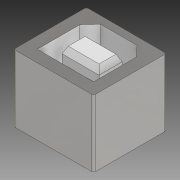
# Autodesk Inventor part: USB B Female Port
Saved by Autodesk Inventor 2016 (Build 200138000, 138)
## iProperties
Created: 2017-10-16
Part Number: USB B Female Port
Material: Steel, Mild
Document SubType Name: Modeling
Designer: admin
Density: 7.85 g/cm^3
Appearance: Semi-Polished
Author: admin
Autodesk Inventor part; units mm, degrees
ref_plane "YZ Plane" through (0, 0, 0) normal (1, 0, 0) x (0, 1, 0)
ref_plane "XZ Plane" through (0, 0, 0) normal (0, 1, 0) x (-1, 0, 0)
ref_plane "XY Plane" through (0, 0, 0) normal (0, 0, 1) x (1, 0, 0)
sketch "Sketch1" plane through (0, 0, 0) normal (0, 0, 1) x (1, 0, 0)
  line L0 (-6.0434, 5.1689) -> (-6.0434, -5.8039) construction
  line L1 (-6.0434, -5.8039) -> (6.0216, -5.8039) construction
  line L2 (6.0216, -5.8039) -> (6.0216, 5.1689) construction
  line L3 (6.0216, 5.1689) -> (-6.0434, 5.1689) construction
  line L4 (-4.2654, -4.0259) -> (4.2436, -4.0259) construction
  line L5 (-4.2654, 2.4003) -> (-4.2654, -4.0259) construction
  line L6 (-2.7795, 4.0259) -> (-4.2654, 2.4003) construction
  line L7 (2.7577, 4.0259) -> (-2.7795, 4.0259) construction
  line L8 (4.2436, 2.4003) -> (2.7577, 4.0259) construction
  line L9 (4.2436, -4.0259) -> (4.2436, 2.4003) construction
  line L10 (-4.2654, -4.0259) -> (4.2436, -4.0259) construction
  line L11 (4.2436, -4.0259) -> (4.2436, 2.4003) construction
  line L12 (4.2436, 2.4003) -> (2.7577, 4.0259) construction
  line L13 (2.7577, 4.0259) -> (-2.7795, 4.0259) construction
  line L14 (-2.7795, 4.0259) -> (-4.2654, 2.4003) construction
  line L15 (-4.2654, 2.4003) -> (-4.2654, -4.0259) construction
  line L16 (1.9887, -1.7399) -> (2.7831, -1.7399) construction
  line L17 (1.9887, -1.8669) -> (1.9887, -1.7399) construction
  line L18 (1.9887, -1.8669) -> (1.0213, -1.8669) construction
  line L19 (1.0213, -1.8669) -> (1.0213, -1.7399) construction
  line L20 (-1.0213, -1.7399) -> (1.0213, -1.7399) construction
  line L21 (-1.0213, -1.8669) -> (-1.0213, -1.7399) construction
  line L22 (-1.0213, -1.8669) -> (-1.9887, -1.8669) construction
  line L23 (-1.9887, -1.8669) -> (-1.9887, -1.7399) construction
  line L24 (-2.8049, -1.7399) -> (-1.9887, -1.7399) construction
  line L25 (-2.8049, 1.7399) -> (-2.8049, -1.7399) construction
  line L26 (-1.9887, 1.7399) -> (-2.8049, 1.7399) construction
  line L27 (-1.9887, 1.8669) -> (-1.9887, 1.7399) construction
  line L28 (-1.0213, 1.8669) -> (-1.9887, 1.8669) construction
  line L29 (-1.0213, 1.8669) -> (-1.0213, 1.7399) construction
  line L30 (1.0213, 1.7399) -> (-1.0213, 1.7399) construction
  line L31 (1.0213, 1.8669) -> (1.0213, 1.7399) construction
  line L32 (1.9887, 1.8669) -> (1.0213, 1.8669) construction
  line L33 (1.9887, 1.8669) -> (1.9887, 1.7399) construction
  line L34 (2.7831, 1.7399) -> (1.9887, 1.7399) construction
  line L35 (2.7831, -1.7399) -> (2.7831, 1.7399) construction
  line L36 (2.1481, -1.1049) -> (2.1481, 1.1049) construction
  line L37 (2.1481, 1.1049) -> (-2.1699, 1.1049) construction
  line L38 (-2.1699, 1.1049) -> (-2.1699, -1.1049) construction
  line L39 (-2.1699, -1.1049) -> (2.1481, -1.1049) construction
  line L40 (-2.8049, 0) -> (2.7831, 0) construction
  line L41 (0, 1.7399) -> (0, -1.7399) construction
  point P0 (0, 0)
  point P1 (0, 0)
  constraints: 84 end point, 5 midpoint
sketch "Sketch2" plane through (0, 0, 0) normal (0, 0, 1) x (1, 0, 0)
  line L0 (6.0216, 5.1689) -> (-6.0434, 5.1689) projected
  line L1 (-6.0434, 5.1689) -> (-6.0434, -5.8039) projected
  line L2 (-6.0434, -5.8039) -> (6.0216, -5.8039) projected
  line L3 (6.0216, -5.8039) -> (6.0216, 5.1689) projected
  line L4 (-4.2654, -4.0259) -> (4.2436, -4.0259) projected
  line L5 (4.2436, -4.0259) -> (4.2436, 2.4003) projected
  line L6 (4.2436, 2.4003) -> (2.7577, 4.0259) projected
  line L7 (2.7577, 4.0259) -> (-2.7795, 4.0259) projected
  line L8 (-2.7795, 4.0259) -> (-4.2654, 2.4003) projected
  line L9 (-4.2654, 2.4003) -> (-4.2654, -4.0259) projected
  point P0 (0, 0)
extrude "Extrusion1" add sketch "Sketch2" along normal blind 9.11
sketch "Sketch3" plane through (0, 0, 0) normal (0, 0, -1) x (-1, 0, 0)
  line L0 (-6.0216, 5.1689) -> (6.0434, 5.1689) projected
  line L1 (6.0434, 5.1689) -> (6.0434, -5.8039) projected
  line L2 (6.0434, -5.8039) -> (-6.0216, -5.8039) projected
  line L3 (-6.0216, -5.8039) -> (-6.0216, 5.1689) projected
  point P0 (0, 0)
extrude "Extrusion2" add sketch "Sketch3" along normal blind 1
sketch "Sketch4" plane through (0, 0, 0) normal (0, 0, 1) x (1, 0, 0)
  line L0 (-1.9887, 1.7399) -> (-2.8049, 1.7399) construction
  line L1 (-2.8049, 1.7399) -> (-2.8049, -1.7399) construction
  line L2 (1.9887, -1.7399) -> (2.7831, -1.7399) construction
  line L3 (2.7831, -1.7399) -> (2.7831, 1.7399) construction
  line L4 (-2.8049, 1.7399) -> (2.7831, 1.7399)
  line L5 (2.7831, 1.7399) -> (2.7831, -1.7399)
  line L6 (2.7831, -1.7399) -> (-2.8049, -1.7399)
  line L7 (-2.8049, -1.7399) -> (-2.8049, 1.7399)
  point P0 (0, 0)
  constraints: 8 end point, 2 parallel, 1 horizontal, 1 perpendicular
extrude "Extrusion3" add sketch "Sketch4" along normal blind 8.11
sketch "Sketch5" plane through (0, 0, 8.11) normal (0, 0, 1) x (1, 0, 0)
  line L0 (2.7831, 1.7399) -> (-2.8049, 1.7399) projected
  line L1 (-2.8049, 1.7399) -> (-2.8049, -1.7399) projected
  line L2 (-2.8049, -1.7399) -> (2.7831, -1.7399) projected
  line L3 (2.7831, -1.7399) -> (2.7831, 1.7399) projected
  point P0 (0, 0)
extrude "Extrusion4" add sketch "Sketch5" along normal blind 1 draft -25
sketch "Sketch6" plane through (0, 0, 0) normal (0, 0, 1) x (1, 0, 0)
  line L0 (-1.0213, 1.8669) -> (-1.9887, 1.8669) construction
  line L1 (1.9887, 1.8669) -> (1.0213, 1.8669) construction
  line L2 (1.9887, -1.8669) -> (1.0213, -1.8669) construction
  line L3 (-1.0213, -1.8669) -> (-1.9887, -1.8669) construction
  line L4 (-1.9887, 1.8669) -> (-1.0213, 1.8669)
  line L5 (-1.0213, 1.8669) -> (-1.0213, 1.7421)
  line L6 (-1.0213, 1.7421) -> (-1.9887, 1.7421)
  line L7 (-1.9887, 1.7421) -> (-1.9887, 1.8669)
  line L8 (1.0213, 1.8669) -> (1.9887, 1.8669)
  line L9 (1.9887, 1.8669) -> (1.9887, 1.7421)
  line L10 (1.9887, 1.7421) -> (1.0213, 1.7421)
  line L11 (1.0213, 1.7421) -> (1.0213, 1.8669)
  line L12 (-1.9887, -1.8669) -> (-1.0213, -1.8669)
  line L13 (-1.0213, -1.8669) -> (-1.0213, -1.7274)
  line L14 (-1.0213, -1.7274) -> (-1.9887, -1.7274)
  line L15 (-1.9887, -1.7274) -> (-1.9887, -1.8669)
  line L16 (1.0213, -1.8669) -> (1.9887, -1.8669)
  line L17 (1.9887, -1.8669) -> (1.9887, -1.7274)
  line L18 (1.9887, -1.7274) -> (1.0213, -1.7274)
  line L19 (1.0213, -1.7274) -> (1.0213, -1.8669)
  point P0 (0, 0)
  constraints: 32 end point, 8 parallel, 4 horizontal, 4 perpendicular, 4 point on line
extrude "Extrusion5" add sketch "Sketch6" along normal blind 6.84
fillet "Fillet1" radius 0.3 4 edges at (6.0216, 5.1689, 4.055) (6.0216, -5.8039, 4.055) (-6.0434, -5.8039, 4.055) (-6.0434, 5.1689, 4.055)
body "Solid1"
